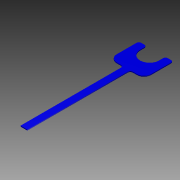
# Autodesk Inventor part: ASAP_Handle_Fixture_New2_1
Saved by Autodesk Inventor 2011 SP2 (Build 150309200, 309)
## iProperties
Created: 2013-02-14
Part Number: ASAP_Handle_Fixture_New2_1
Document SubType Name: Modeling
Designer: sungwook
Density: 1 g/cm^3
Author: sungwook
Autodesk Inventor part; units mm, degrees
ref_plane "YZ Plane" through (0, 0, 0) normal (1, 0, 0) x (0, 1, 0)
ref_plane "XZ Plane" through (0, 0, 0) normal (0, 1, 0) x (-1, 0, 0)
ref_plane "XY Plane" through (0, 0, 0) normal (0, 0, 1) x (1, 0, 0)
sketch "Sketch1" plane through (0, 0, 0) normal (0, 0, 1) x (1, 0, 0)
  line L0 (0, -78.4) -> (0, 29.4) projected
  line L1 (5.5, 10.25) -> (5.5, 14)
  line L2 (5.5, 14) -> (10, 14)
  line L3 (10, 14) -> (10, -3)
  line L4 (10, -3) -> (2, -3)
  line L5 (2, -3) -> (2, -63)
  line L6 (2, -63) -> (0, -63)
  line L7 (-5.5, 10.25) -> (-5.5, 14)
  line L8 (-5.5, 14) -> (-10, 14)
  line L9 (-10, 14) -> (-10, -3)
  line L10 (-10, -3) -> (-2, -3)
  line L11 (-2, -3) -> (-2, -63)
  line L12 (-2, -63) -> (0, -63)
  arc A0 (-5.5, 10.25) -> (5.5, 10.25) centre (0, 10.25) ccw
  point P0 (0, 0)
  point P1 (5.5, 3.5)
  point P2 (-5.5, 3.5)
  point P3 (5.5, -3)
  point P4 (0, 14)
  dimension "d0" = 4.5
  dimension "d1" = 20
  dimension "d2" = 4
  dimension "d7" = 60
  dimension "d13" = 11
  dimension "d14" = 17
  dimension "d16" = 3.75
  constraints: 24 end point, 5 point on line, 5 symmetric about line, 2 perpendicular, 2 point on circle, 1 centre point, 1 parallel
  measures "d0" distance of L2.end L1.end
  measures "d1" distance between parallel lines of L3 L9
  measures "d2" distance between parallel lines of L5 L11
  measures "d7" distance from line of L5.end L4
  measures "d13" diameter of A0
  measures "d14" distance between parallel lines of L10 L8
  measures "d16" distance of A0.centre point (0, 14)
extrude "Extrusion1" add sketch "Sketch1" along normal blind 0.508
fillet "Fillet1" radius 1.25 4 edges at (-10, 14, 0.254) (10, 14, 0.254) (-5.5, 14, 0.254) (5.5, 14, 0.254)
fillet "Fillet3" radius 4 2 edges at (-10, -3, 0.254) (10, -3, 0.254)
fillet "Fillet4" radius 1.5 2 edges at (-2, -3, 0.254) (2, -3, 0.254)
body "Solid1"
